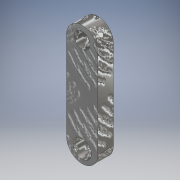
# Autodesk Inventor part: reverse gear drag link
Saved by Autodesk Inventor 2017 (Build 210142000, 142)
## iProperties
Created: 2018-11-03
Part Number: reverse gear drag link
Material: Generic
Document SubType Name: Modeling
Designer: User
Density: 1 g/cm^3
Appearance: Default
Author: User
Autodesk Inventor part; units mm, degrees
ref_plane "YZ Plane" through (0, 0, 0) normal (1, 0, 0) x (0, 1, 0)
ref_plane "XZ Plane" through (0, 0, 0) normal (0, 1, 0) x (-1, 0, 0)
ref_plane "XY Plane" through (0, 0, 0) normal (0, 0, 1) x (1, 0, 0)
sketch "Sketch1" plane through (0, 0, 0) normal (0, 1, 0) x (-1, 0, 0)
  line L0 (0, 0) -> (6, 0)
  line L1 (6, 0) -> (6, -23)
  line L2 (6, -23) -> (0, -23)
  line L3 (0, -23) -> (0, 0)
  circle A0 centre (3, -2.5) radius 1.5
  circle A1 centre (3, -20.5) radius 1.75
  dimension "d0" = 6
  dimension "d1" = 23
  dimension "d2" = 6
  dimension "d4" = 3
  dimension "d5" = 3.5
  dimension "d6" = 2.5
  dimension "d7" = 2.5
  constraints: 8 end point, 2 centre point, 2 horizontal, 1 perpendicular
  measures "d0" distance of L0.start L0.end
  measures "d1" distance of L0.end L1.end
  measures "d2" distance of L1.end L2.end
  measures "d4" diameter of A0
  measures "d5" diameter of A1
  measures "d6" distance from line of L0 A0.centre
  measures "d7" distance from line of L2 A1.centre
extrude "Extrusion1" add sketch "Sketch1" along normal blind 3
fillet "Fillet1" radius 3 1 edges at (-6, 1.5, 0)
fillet "Fillet2" radius 3 3 edges at (0, 1.5, 0) (-6, 1.5, -23) (0, 1.5, -23)
body "Solid1"
